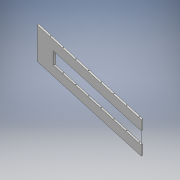
# Autodesk Inventor part: sidesupport
Saved by Autodesk Inventor 2017 (Build 210142000, 142)
## iProperties
Created: 2016-12-06
Part Number: sidesupport
Material: Generic
Document SubType Name: Sheet Metal
Designer: aesen
Density: 1 g/cm^3
Sheet Metal Rule: Default_mm
Appearance: Default
Author: aesen
Autodesk Inventor part; units mm, degrees
ref_plane "YZ Plane" through (0, 0, 0) normal (1, 0, 0) x (0, 1, 0)
ref_plane "XZ Plane" through (0, 0, 0) normal (0, 1, 0) x (-1, 0, 0)
sketch "Sketch4" plane through (0, 0, 0) normal (0, 0, 1) x (1, 0, 0)
  line L0 (293.2796, 30.0061) -> (-199.5823, 140.5264)
  line L1 (293.2796, 36.3718) -> (-199.5823, 146.9202)
  line L2 (-199.5823, 146.9202) -> (-199.5823, 140.5264)
  line L3 (293.2796, 30.0061) -> (-199.5823, 140.5264)
  line L4 (293.2796, 36.3718) -> (-199.5823, 146.9202)
  line L5 (-199.5823, 146.9202) -> (-199.5823, 140.5264)
  line L6 (293.2796, 30.0061) -> (293.2796, 36.3718)
  constraints: 14 end point
sketch "Sketch5" plane through (0, 0, 0) normal (0, 0, 1) x (1, 0, 0)
  circle A0 centre (280.3828, 36.0784) radius 3.5
  circle A1 centre (220.3828, 49.5364) radius 3.5
  circle A2 centre (160.3828, 62.9943) radius 3.5
  circle A3 centre (100.3828, 76.4523) radius 3.5
  circle A4 centre (40.3604, 89.9135) radius 3.5
  circle A5 centre (-139.6396, 130.2873) radius 3.5
  circle A6 centre (-79.6396, 116.8294) radius 3.5
  circle A7 centre (-19.6396, 103.3714) radius 3.5
  constraints: 8 centre point
extrude "Extrusion3" add sketch "Sketch4" along normal blind 115.75
ref_plane "Work Plane3" through (111499.6524, -24907.1137, 0) normal (-0.2188346, -0.975762, 0) x (0, 0, -1)
sketch "Sketch6" plane through (111499.6524, -24907.1137, 0) normal (-0.2188346, -0.975762, 0) x (0, 0, -1)
  line L0 (0, -114474.0796) -> (-115.4577, -114474.0796)
  line L1 (-115.4577, -114474.0796) -> (-115.4577, -113968.0685)
  line L2 (-115.4577, -113968.0685) -> (0, -113968.0685)
  line L3 (0, -113968.0685) -> (0, -114474.0796)
  line L4 (0, -113968.0539) -> (-115.75, -113968.0539) projected
  line L5 (-27.7607, -113968.0539) -> (-91.2309, -113968.0539)
  line L6 (-75.4577, -113983.6101) -> (-36.9803, -113983.6101)
  line L7 (-35, -113968.0685) -> (-80.4577, -113968.0685)
  line L8 (-80.4577, -113968.0685) -> (-80.4577, -114394.0796)
  line L9 (-80.4577, -114394.0796) -> (-35, -114394.0796)
  line L10 (-35, -114394.0796) -> (-35, -113968.0685)
  point P0 (0, -114247.6585)
  dimension "d28" = 506.0111
  dimension "d29" = 115.4577
  dimension "d30" = 35
  dimension "d32" = 80
  dimension "d42" = 35
  constraints: 20 end point, 4 parallel, 3 horizontal, 2 perpendicular, 2 point on line
  measures "d28" distance of L2.end L0.start
  measures "d29" distance of L1.end L2.end
  measures "d30" distance between parallel lines of L10 L3
  measures "d32" distance between parallel lines of L9 L0
  measures "d42" distance between parallel lines of L8 L1
emboss "Emboss1" sketch "Sketch6" operation cut depth 8 direction (-0.2188346, -0.975762, 0) contours L10 L9 L8 L2
hole "Hole1" at (-139.6396, 130.2873, 0) at (-79.6396, 116.8294, 0) at (-19.6396, 103.3714, 0) at (40.3604, 89.9135, 0) at (100.3828, 76.4523, 0) at (160.3828, 62.9943, 0) at (220.3828, 49.5364, 0) at (280.3828, 36.0784, 0) direction (0, 0, 1) diameter 3 end through all
equation "\"d40\" = Thickness"
equation "\"BendRadius\" = Thickness"
equation "\"BendReliefWidth\" = Thickness"
equation "\"BendReliefDepth\" = 0.5 * Thickness"
equation "\"CornerReliefSize\" = 4 * Thickness"
equation "\"MinimumRemnant\" = 2 * Thickness"
equation "\"TransitionRadius\" = BendRadius"
equation "\"JacobiRadiusSize\" = BendRadius"
equation "\"GapSize\" = Thickness"
equation "\"Thickness\" = 0.5"
body "Solid3"
